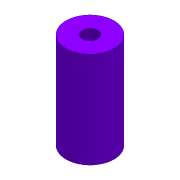
# Autodesk Inventor part: Solenoid600
Saved by Autodesk Inventor 2022.2 (Build 262287010, 287A)
## iProperties
RuleStatus: InUse
Created: 2021-04-26
Part Number: Solenoid600
Material: Generic
Document SubType Name: Modeling
Designer: Josep
Density: 1 g/cm^3
Appearance: Solenoid
Mass: 26436.5 g
Surface Area: 7101.57 cm^2
Volume: 26436.5 cm^3
Author: Josep
Autodesk Inventor part; units mm, degrees
ref_plane "YZ Plane" through (0, 0, 0) normal (1, 0, 0) x (0, 1, 0)
ref_plane "XZ Plane" through (0, 0, 0) normal (0, 1, 0) x (-1, 0, 0)
ref_plane "XY Plane" through (0, 0, 0) normal (0, 0, 1) x (1, 0, 0)
sketch "Sketch1" plane through (0, 0, 0) normal (0, 0, 1) x (1, 0, 0)
  circle A0 centre (0, 0) radius 125
  circle A1 centre (0, 0) radius 40
  dimension "d6" = 250
  dimension "d9" = 80
  constraints: 2 centre point, 2 coincident
  measures "d6" diameter of A0
  measures "d9" diameter of A1
extrude "Extrusion1" add sketch "Sketch1" along normal mid plane 500
equation "\"d7\" = Length"
equation "\"Length\" = 500"
body "Solid1"
